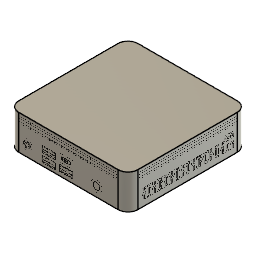
GB-BRR5-4500 (Autodesk Fusion 360 design; units mm, degrees)
Autodesk Fusion 360 part; units mm, degrees
sketch "Sketch1" plane through (0, 0, 0) normal (0, 1, 0) x (1, 0, 0)
  line L0 (59.75, -59.75) -> (-59.75, -59.75)
  line L1 (-59.75, -59.75) -> (-59.75, 59.75)
  line L2 (-59.75, 59.75) -> (59.75, 59.75)
  line L3 (59.75, 59.75) -> (59.75, -59.75)
  line L4 (59.75, -59.75) -> (-59.75, 59.75) construction
  line L5 (-59.75, -59.75) -> (59.75, 59.75) construction
  dimension "d2" = 119.5
  constraint horizontal L0
  constraint perpendicular L0 L1
  constraint parallel L0 L2
  constraint parallel L1 L3
  constraint coincident L4 origin
  constraint coincident L5 origin
  constraint equal L0 L1
  measures "d2" distance of L0 L2
extrude "Extrude1" add sketch "Sketch1" along normal blind 34.7
fillet "Fillet1" radius 10 4 edges at (-59.75, 17.35, 59.75) (59.75, 17.35, 59.75) (-59.75, 17.35, -59.75) (59.75, 17.35, -59.75)
sketch "Sketch4" plane through (0, 0, 0) normal (0, -1, 0) x (1, 0, 0)
  line L0 (-49.75, -59.75) -> (49.75, -59.75)
  line L1 (59.75, -49.75) -> (59.75, 49.75)
  line L2 (49.75, 59.75) -> (-49.75, 59.75)
  line L3 (-59.75, 49.75) -> (-59.75, -49.75)
  line L4 (-49.4, 45.1) -> (-38.4, 45.1)
  arc A0 (-38.4, 45.1) -> (-38.4, 53.5) centre (-38.4, 49.3) ccw
  line L5 (-38.4, 53.5) -> (-49.4, 53.5)
  arc A1 (-49.4, 53.5) -> (-49.4, 45.1) centre (-49.4, 49.3) ccw
  line L6 (-49.4, 49.3) -> (-38.4, 49.3) construction
  line L7 (-49.4, -53.7) -> (-38.4, -53.7)
  arc A2 (-38.4, -53.7) -> (-38.4, -45.3) centre (-38.4, -49.5) ccw
  line L8 (-38.4, -45.3) -> (-49.4, -45.3)
  arc A3 (-49.4, -45.3) -> (-49.4, -53.7) centre (-49.4, -49.5) ccw
  line L9 (-49.4, -49.5) -> (-38.4, -49.5) construction
  line L10 (49.1, -45.3) -> (38.1, -45.3)
  arc A4 (38.1, -45.3) -> (38.1, -53.7) centre (38.1, -49.5) ccw
  line L11 (38.1, -53.7) -> (49.1, -53.7)
  arc A5 (49.1, -53.7) -> (49.1, -45.3) centre (49.1, -49.5) ccw
  line L12 (49.1, -49.5) -> (38.1, -49.5) construction
  line L13 (37.35, 45.1) -> (48.35, 45.1)
  arc A6 (48.35, 45.1) -> (48.35, 53.5) centre (48.35, 49.3) ccw
  line L14 (48.35, 53.5) -> (37.35, 53.5)
  arc A7 (37.35, 53.5) -> (37.35, 45.1) centre (37.35, 49.3) ccw
  line L15 (37.35, 49.3) -> (48.35, 49.3) construction
  arc A8 (49.75, -59.75) -> (59.75, -49.75) centre (49.75, -49.75) ccw
  arc A9 (59.75, 49.75) -> (49.75, 59.75) centre (49.75, 49.75) ccw
  arc A10 (-49.75, 59.75) -> (-59.75, 49.75) centre (-49.75, 49.75) ccw
  arc A11 (-59.75, -49.75) -> (-49.75, -59.75) centre (-49.75, -49.75) ccw
  dimension "d6" = 4.2
  dimension "d7" = 11
  dimension "d8" = 49.4
  dimension "d9" = 49.3
  dimension "d14" = 37.35
  dimension "d15" = 49.5
  dimension "d16" = 49.1
  constraint tangent L4 A0
  constraint tangent A0 L5
  constraint parallel L4 L5
  constraint tangent L5 A1
  constraint tangent L4 A1
  constraint horizontal L6
  constraint tangent L7 A2
  constraint tangent A2 L8
  constraint parallel L7 L8
  constraint tangent L8 A3
  constraint tangent L7 A3
  constraint parallel L0 L9
  constraint tangent L10 A4
  constraint tangent A4 L11
  constraint parallel L10 L11
  constraint tangent L11 A5
  constraint tangent L10 A5
  constraint perpendicular L1 L12
  constraint tangent L13 A6
  constraint tangent A6 L14
  constraint parallel L13 L14
  constraint tangent L14 A7
  constraint tangent L13 A7
  constraint parallel L10 L15
  constraint coincident L6 A7.centre
  constraint vertical A1.centre A3.centre
  constraint equal L6 L9
  constraint equal L9 L12
  constraint equal L12 L15
  constraint equal A0 A5
  constraint equal A0 A2
  constraint equal A0 A7
  constraint coincident L9 A4.centre
  measures "d6" radius of A0
  measures "d7" distance of A1.centre A0.centre
  measures "d8" horizontal distance of origin A1.centre
  measures "d9" distance of origin L6
  measures "d14" horizontal distance of origin A7.centre
  measures "d15" distance of origin L9
  measures "d16" horizontal distance of origin A5.centre
extrude "Extrude2" add sketch "Sketch4" along normal blind 2.5 contours L4 A0 L5 A1 | L7 A2 L8 A3 | L10 A4 L11 A5 | L13 A6 L14 A7
sketch "Sketch5" plane through (0, 0, 0) normal (0, -1, 0) x (1, 0, 0)
  line L0 (37.35, 53.5) -> (48.35, 53.5)
  arc A0 (48.35, 45.1) -> (48.35, 53.5) centre (48.35, 49.3) ccw
  line L1 (48.35, 45.1) -> (37.35, 45.1)
  arc A1 (37.35, 53.5) -> (37.35, 45.1) centre (37.35, 49.3) ccw
  line L2 (-49.4, 53.5) -> (-38.4, 53.5)
  arc A2 (-38.4, 45.1) -> (-38.4, 53.5) centre (-38.4, 49.3) ccw
  line L3 (-38.4, 45.1) -> (-49.4, 45.1)
  arc A3 (-49.4, 53.5) -> (-49.4, 45.1) centre (-49.4, 49.3) ccw
  line L4 (49.1, -53.7) -> (38.1, -53.7)
  arc A4 (38.1, -45.3) -> (38.1, -53.7) centre (38.1, -49.5) ccw
  line L5 (38.1, -45.3) -> (49.1, -45.3)
  arc A5 (49.1, -53.7) -> (49.1, -45.3) centre (49.1, -49.5) ccw
  line L6 (-49.4, -45.3) -> (-38.4, -45.3)
  arc A6 (-38.4, -53.7) -> (-38.4, -45.3) centre (-38.4, -49.5) ccw
  line L7 (-38.4, -53.7) -> (-49.4, -53.7)
  arc A7 (-49.4, -45.3) -> (-49.4, -53.7) centre (-49.4, -49.5) ccw
  line L8 (-49.75, -59.75) -> (49.75, -59.75)
  line L9 (59.75, -49.75) -> (59.75, 49.75)
  line L10 (49.75, 59.75) -> (-49.75, 59.75)
  line L11 (-59.75, 49.75) -> (-59.75, -49.75)
  line L12 (-40, 0) -> (40, 0) construction
  circle A8 centre (-40, 0) radius 1.25
  circle A9 centre (40, 0) radius 1.25
  arc A10 (49.75, -59.75) -> (59.75, -49.75) centre (49.75, -49.75) ccw
  arc A11 (59.75, 49.75) -> (49.75, 59.75) centre (49.75, 49.75) ccw
  arc A12 (-49.75, 59.75) -> (-59.75, 49.75) centre (-49.75, 49.75) ccw
  arc A13 (-59.75, -49.75) -> (-49.75, -59.75) centre (-49.75, -49.75) ccw
  dimension "d17" = 2.5
  dimension "d18" = 80
  constraint horizontal L12
  constraint coincident L12.start A8.centre
  constraint coincident L12.end A9.centre
  constraint midpoint origin L12
  constraint equal A8 A9
  measures "d17" diameter of A8
  measures "d18" distance of L12.start L12.end
extrude "Extrude3" cut sketch "Sketch5" against normal blind 3 contours A8 | A9
